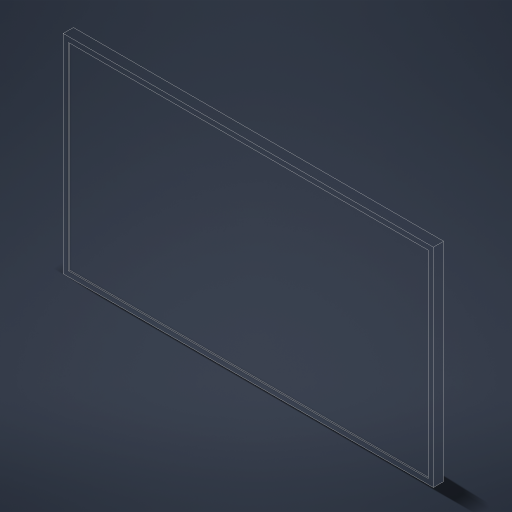
# Autodesk Inventor part: TV 65
Saved by Autodesk Inventor 2024.2 (Build 282272000, 272)
## iProperties
Created: 2025-08-11
Part Number: TV 65
Material: Generic
Document SubType Name: Modeling
Designer: Luca
Density: 1 g/cm^3
Appearance: Glossy - Black
Author: Luca
Autodesk Inventor part; units mm, degrees
ref_plane "YZ Plane" through (0, 0, 0) normal (1, 0, 0) x (0, 1, 0)
ref_plane "XZ Plane" through (0, 0, 0) normal (0, 1, 0) x (-1, 0, 0)
ref_plane "XY Plane" through (0, 0, 0) normal (0, 0, 1) x (1, 0, 0)
sketch "Sketch1" plane through (0, 0, 0) normal (0, 0, 1) x (1, 0, 0)
  line L0 (-719.5, -404.5) -> (719.5, -404.5)
  line L1 (719.5, -404.5) -> (719.5, 404.5)
  line L2 (719.5, 404.5) -> (-719.5, 404.5)
  line L3 (-719.5, 404.5) -> (-719.5, -404.5)
  line L4 (-719.5, -404.5) -> (719.5, 404.5) construction
  line L5 (719.5, -404.5) -> (-719.5, 404.5) construction
  point P0 (0, 0)
  dimension "d0" = 1439
  dimension "d1" = 809
  constraints: 12 end point, 2 midpoint, 2 parallel, 1 horizontal, 1 perpendicular
  measures "d0" distance of L2.end L1.end
  measures "d1" distance of L1.end L0.end
extrude "Extrusion1" add sketch "Sketch1" along normal blind 60
shell "Shell1" thickness 20 removed faces 1 at (-239.8333, 134.8333, 60) ; own thickness 55 on faces at (-239.8333, 134.8333, 0)
chamfer "Chamfer1" distance 20 angle 45 4 edges at (719.5, 0, 0) (0, 404.5, 0) (-719.5, 0, 0) (0, -404.5, 0)
body "Solid1"
